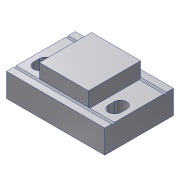
# Autodesk Inventor part: Holding Block
Saved by Autodesk Inventor 2016 (Build 200138000, 138)
## iProperties
Created: 2015-08-18
Part Number: Holding Block
Material: Aluminum 6061
Document SubType Name: Modeling
Density: 2.7 g/cm^3
Appearance: Aluminum - Flat
Autodesk Inventor part; units mm, degrees
ref_plane "YZ Plane" through (0, 0, 0) normal (1, 0, 0) x (0, 1, 0)
ref_plane "XZ Plane" through (0, 0, 0) normal (0, 1, 0) x (-1, 0, 0)
ref_plane "XY Plane" through (0, 0, 0) normal (0, 0, 1) x (1, 0, 0)
sketch "Sketch1" plane through (0, 0, 0) normal (1, 0, 0) x (0, 1, 0)
  line L0 (4.25, 20) -> (30.75, 20)
  line L1 (30.75, 20) -> (30.75, 12)
  line L2 (30.75, 12) -> (35, 12)
  line L3 (35, 12) -> (35, 0)
  line L4 (35, 0) -> (16.25, 0)
  line L5 (16.25, 0) -> (16.25, -5)
  line L6 (16.25, -5) -> (8.75, -5)
  line L7 (8.75, -5) -> (8.75, 0)
  line L8 (8.75, 0) -> (0, 0)
  line L9 (0, 0) -> (0, 12)
  line L10 (0, 12) -> (4.25, 12)
  line L11 (4.25, 12) -> (4.25, 20)
  line L12 (3.5429, 12) -> (4.25, 12.7071)
  line L13 (4.25, 12.7071) -> (4.9571, 12)
  line L14 (4.9571, 12) -> (4.25, 11.2929)
  line L15 (4.25, 11.2929) -> (3.5429, 12)
  line L16 (30.75, 12.7071) -> (31.4571, 12)
  line L17 (31.4571, 12) -> (30.75, 11.2929)
  line L18 (30.75, 11.2929) -> (30.0429, 12)
  line L19 (30.0429, 12) -> (30.75, 12.7071)
  dimension "d0" = 35
  dimension "d3" = 7.5
  dimension "d4" = 8
  dimension "d5" = 25
  dimension "d6" = 5
  dimension "d7" = 22
  dimension "d9" = 12
  dimension "d11" = 4.25
  dimension "d12" = 4.25
  dimension "d19" = 1
  dimension "d20" = 0.5
  dimension "d21" = 0.5
  dimension "d22" = 1
  dimension "d23" = 45
  constraints: 40 end point, 10 perpendicular, 8 point on line, 5 parallel, 1 coincident, 1 collinear, 1 horizontal, 1 vertical
  measures "d0" distance between parallel lines of L9 L3
  measures "d3" distance of L5.end L6.end
  measures "d4" distance between parallel lines of L10 L0
  measures "d5" distance between parallel lines of L6 L0
  measures "d6" distance between parallel lines of L8 L6
  measures "d7" distance between parallel lines of L1 L7
  measures "d9" distance between parallel lines of L5 L11
  measures "d11" distance between parallel lines of L9 L11
  measures "d12" distance of L1.end L2.end
  measures "d19" distance between parallel lines of L15 L13
  measures "d20" distance from line of L10.end L14
  measures "d21" distance from line of L1.end L18
  measures "d22" distance between parallel lines of L17 L19
  measures "d23" angle of L10 L13
extrude "Extrusion1" add sketch "Sketch1" along normal mid plane 50 contours L0 L1 L19 L18 L17 L2 L3 L4 L5 L6 L7 L8 L9 L10 L15 L14 L13 L11
sketch "Sketch2" plane through (-25, 0, 0) normal (0, -1, 0) x (1, 0, 0)
  line L0 (0, 20) -> (12.5, 20)
  line L1 (12.5, 20) -> (12.5, 12)
  line L2 (12.5, 12) -> (0, 12)
  line L3 (0, 12) -> (0, 20)
  line L4 (37.5, 20) -> (50, 20)
  line L5 (50, 20) -> (50, 12)
  line L6 (50, 12) -> (37.5, 12)
  line L7 (37.5, 12) -> (37.5, 20)
  line L8 (50, -5) -> (35, -5)
  line L9 (35, -5) -> (35, 0)
  line L10 (35, 0) -> (50, 0)
  line L11 (50, 0) -> (50, -5)
  line L12 (0, -5) -> (15, -5)
  line L13 (15, -5) -> (15, 0)
  line L14 (15, 0) -> (0, 0)
  line L15 (0, 0) -> (0, -5)
  line L16 (0, -5) -> (50, -5) projected
  line L17 (50, 0) -> (50, -5) projected
  line L18 (50, 20) -> (0, 20) projected
  line L19 (0, 12.7071) -> (0, 20) projected
  line L20 (0, 12) -> (50, 12) projected
  line L21 (25, 0) -> (50, 0) projected
  dimension "d15" = 25
  dimension "d16" = 20
  constraints: 32 end point, 8 collinear, 8 parallel, 6 point on line, 4 horizontal, 4 perpendicular
  measures "d15" distance between parallel lines of L7 L1
  measures "d16" distance between parallel lines of L9 L13
extrude "Extrusion2" cut sketch "Sketch2" against normal through all contours L0 L1 L2 L3 | L4 L5 L6 L7 | L12 L15 L14 L13 | L8 L9 L10 L11
sketch "Sketch4" plane through (12.5, 30.0429, 12) normal (0, 0, 1) x (1, 0, 0)
  line L0 (-31.5, -19.0429) -> (-31.5, -16.0429) construction
  line L1 (-28.25, -19.0429) -> (-28.25, -16.0429)
  line L2 (-34.75, -16.0429) -> (-34.75, -19.0429)
  arc A0 (-34.75, -19.0429) -> (-28.25, -19.0429) centre (-31.5, -19.0429) ccw
  arc A1 (-28.25, -16.0429) -> (-34.75, -16.0429) centre (-31.5, -16.0429) ccw
  line L3 (-37.5, -25.0858) -> (-37.5, 0) projected
  line L4 (-22.5, -21.2929) -> (-2.5, -21.2929) projected
  point P0 (-31.5, -17.5429)
  dimension "d24" = 6.5
  dimension "d25" = 3
  dimension "d26" = 6
  dimension "d27" = 3.75
  constraints: 8 end point, 4 point on circle, 4 tangent, 2 centre point, 1 midpoint, 1 parallel, 1 vertical
  measures "d24" distance between parallel lines of L1 L2
  measures "d25" distance of L0.start L0.end
  measures "d26" distance from line of L3 point (-31.5, -17.543)
  measures "d27" distance from line of L4 point (-31.5, -17.543)
extrude "Extrusion3" cut sketch "Sketch4" against normal through all
mirror "Mirror1" about plane through (0, 0, 0) normal (1, 0, 0) of "Extrusion3"
equation "\"d21\" = d20"
equation "\"d22\" = d19"
equation "\"d27\" = 0.5 * d3"
body "Solid1"
